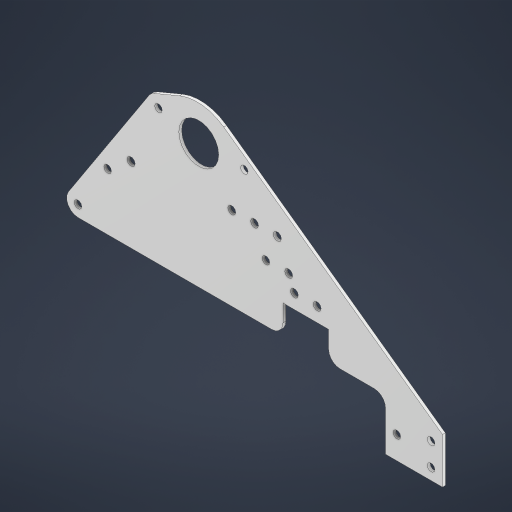
# Autodesk Inventor part: plate_mid
Saved by Autodesk Inventor 2024 (Build 280153000, 153)
## iProperties
Created: 2023-11-09
Part Number: plate_mid
Material: Acetal Resin, White
Document SubType Name: Modeling
Designer: avere
Density: 1.425 g/cm^3
Appearance: Smooth - White
Author: avere
Autodesk Inventor part; units mm, degrees
ref_plane "YZ Plane" through (0, 0, 0) normal (1, 0, 0) x (0, 1, 0)
ref_plane "XZ Plane" through (0, 0, 0) normal (0, 1, 0) x (-1, 0, 0)
ref_plane "XY Plane" through (0, 0, 0) normal (0, 0, 1) x (1, 0, 0)
sketch "Sketch1" plane through (0, 0, 0) normal (0, 0, 1) x (1, 0, 0)
  line L0 (177.2398, 109.2972) -> (163.051, 103.3471)
  line L1 (323.85, -6.35) -> (323.85, 19.05)
  line L2 (323.85, -6.35) -> (292.1, -6.35)
  line L3 (292.1, -6.35) -> (292.1, 15.875)
  line L4 (292.1, -6.35) -> (323.85, -6.35)
  arc A0 (292.1, 15.875) -> (285.75, 22.225) centre (285.75, 15.875) ccw
  circle A1 centre (317.5, 0) radius 2.0955
  circle A2 centre (317.5, 12.7) radius 2.0955
  line L5 (120.65, 22.225) -> (184.15, 22.225)
  circle A3 centre (298.45, 6.35) radius 2.0955
  arc A4 (201.8633, 106.5157) -> (177.2398, 109.2972) centre (187.0626, 85.8735) ccw
  circle A5 centre (187.9687, 91.7095) radius 11.1125
  line L6 (260.35, 28.575) -> (260.35, 38.1)
  line L7 (260.35, 38.1) -> (234.95, 38.1)
  line L8 (234.95, 38.1) -> (234.95, 28.575)
  line L9 (184.15, 22.225) -> (228.6, 22.225)
  line L10 (266.7, 22.225) -> (285.75, 22.225)
  arc A6 (228.6, 22.225) -> (234.95, 28.575) centre (228.6, 28.575) ccw
  arc A7 (260.35, 28.575) -> (266.7, 22.225) centre (266.7, 28.575) ccw
  line L11 (115.328, 32.039) -> (160.1848, 100.9551)
  circle A8 centre (150.2443, 64.09) radius 2.2479
  circle A9 centre (225.425, 53.975) radius 2.0955
  circle A10 centre (238.125, 53.975) radius 2.1844
  line L12 (323.85, 19.05) -> (291.7679, 42.0532)
  line L13 (323.85, 19.05) -> (201.8633, 106.5157)
  circle A11 centre (241.3, 46.0375) radius 2.1844
  circle A12 centre (254, 46.0375) radius 2.1844
  circle A13 centre (206.375, 68.6706) radius 2.1844
  circle A14 centre (219.075, 68.6706) radius 2.1844
  circle A15 centre (231.775, 68.6706) radius 2.2479
  circle A16 centre (213.3687, 91.7095) radius 2.0955
  circle A17 centre (120.65, 28.575) radius 2.0955
  circle A18 centre (165.5067, 97.4911) radius 2.0955
  arc A19 (115.328, 32.039) -> (120.65, 22.225) centre (120.65, 28.575) ccw
  arc A20 (163.051, 103.3471) -> (160.1848, 100.9551) centre (165.5067, 97.4911) ccw
  circle A21 centre (137.1826, 53.975) radius 2.0955
  point P0 (292.1, 22.225)
  point P1 (146.05, 22.225)
  point P2 (260.35, 22.225)
  point P3 (124.6512, 46.3627)
  point P4 (148.9618, 83.7126)
  dimension "d14" = 31.75
  dimension "d15" = 28.575
  dimension "d16" = 6.35
  dimension "d18" = 4.191
  dimension "d19" = 4.191
  dimension "d29" = 4.191
  dimension "d30" = 25.4
  dimension "d32" = 22.225
  dimension "d37" = 15.875
  dimension "d38" = 6.35
  dimension "d60" = 4.4958
  dimension "d69" = 4.3688
  dimension "d78" = 4.3688
  dimension "d79" = 4.3688
  dimension "d97" = 4.191
  dimension "d105" = 12.7
  dimension "d106" = 12.7
  dimension "d107" = 4.191
  constraints: 28 end point, 22 centre point, 15 tangent, 12 point on circle, 6 point on line, 4 perpendicular, 2 coincident, 2 horizontal, 1 equal radius, 1 vertical, 3 other
  measures "d14" distance of L1.start L2.end
  measures "d15" distance of L2.end point (292.1, 22.225)
  measures "d16" radius of A0
  measures "d18" diameter of A1
  measures "d19" diameter of A2
  measures "d29" diameter of A3
  measures "d30" radius of A4
  measures "d32" diameter of A5
  measures "d37" distance of point (260.35, 22.225) L6.end
  measures "d38" radius of A6
  measures "d60" diameter of A8
  measures "d69" diameter of A10
  measures "d78" diameter of A11
  measures "d79" diameter of A12
  measures "d97" diameter of A16
  measures "d105" diameter of A19
  measures "d106" diameter of A20
  measures "d107" diameter of A21
extrude "Extrusion1" add sketch "Sketch1" along normal blind 1.5875
body "Solid1"
